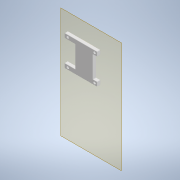
# Autodesk Inventor part: OLED
Saved by Autodesk Inventor 2021 (Build 250183000, 183)
## iProperties
Created: 2022-09-01
Part Number: OLED
Material: Generic
Document SubType Name: Modeling
Designer: cmzgt
Density: 1 g/cm^3
Appearance: Default
Author: cmzgt
Autodesk Inventor part; units mm, degrees
ref_plane "YZ Plane" through (0, 0, 0) normal (1, 0, 0) x (0, 1, 0)
ref_plane "XZ Plane" through (0, 0, 0) normal (0, 1, 0) x (-1, 0, 0)
ref_plane "XY Plane" through (0, 0, 0) normal (0, 0, 1) x (1, 0, 0)
ref_plane "Work Plane1" through (0, 0, 0) normal (0, 0, 1) x (1, 0, 0)
sketch "Sketch1" plane through (0, 0, 0) normal (0, 0, 1) x (1, 0, 0)
  line L0 (26.085, -12.7501) -> (26.085, -38.7501) projected
  line L1 (15.085, -12.7501) -> (26.085, -12.7501) projected
  line L2 (15.085, -38.7501) -> (15.085, -12.7501) projected
  line L3 (26.085, -38.7501) -> (15.085, -38.7501) projected
  line L4 (26.085, -25.7501) -> (15.085, -25.7501)
  line L5 (20.585, -38.7501) -> (20.585, -12.7501)
  line L6 (15.2194, -38.2641) -> (25.9506, -38.2641)
  line L7 (25.9506, -38.2641) -> (25.9506, -13.236)
  line L8 (25.9506, -13.236) -> (15.2194, -13.236)
  line L9 (15.2194, -13.236) -> (15.2194, -38.2641)
  line L10 (15.2194, -38.2641) -> (25.9506, -13.236) construction
  line L11 (25.9506, -38.2641) -> (15.2194, -13.236) construction
  point P0 (0, 0)
  point P1 (20.585, -25.7501)
  constraints: 16 end point, 7 midpoint, 2 parallel, 1 horizontal, 1 perpendicular
extrude "Extrusion1" add sketch "Sketch1" against normal blind 1 contours L7 L6 L5 L4 | L4 L5 L8 L7 | L5 L4 L9 L8 | L5 L6 L9 L4
sketch "Sketch2" plane through (0, 0, 0) normal (0, 0, 1) x (1, 0, 0)
  line L0 (15.2194, -13.236) -> (15.2194, -38.2641) projected
  line L1 (15.2194, -38.2641) -> (25.9506, -38.2641) projected
  line L2 (25.9506, -38.2641) -> (25.9506, -13.236) projected
  line L3 (25.9506, -13.236) -> (15.2194, -13.236) projected
  line L4 (13.1635, -39.268) -> (28.9935, -39.268)
  line L5 (28.9935, -39.268) -> (28.9935, -12.2321)
  line L6 (28.9935, -12.2321) -> (13.1635, -12.2321)
  line L7 (13.1635, -12.2321) -> (13.1635, -39.268)
  line L8 (13.1635, -39.268) -> (28.9935, -12.2321) construction
  line L9 (28.9935, -39.268) -> (13.1635, -12.2321) construction
  line L10 (28.9935, -12.2321) -> (32.8035, -12.2321)
  line L11 (32.8035, -12.2321) -> (32.8035, -16.0421)
  line L12 (32.8035, -16.0421) -> (28.9935, -16.0421)
  line L13 (28.9935, -39.268) -> (32.8035, -39.268)
  line L14 (32.8035, -39.268) -> (32.8035, -35.458)
  line L15 (32.8035, -35.458) -> (28.9935, -35.458)
  line L16 (13.1635, -12.2321) -> (3.8747, -12.2321)
  line L17 (3.8747, -12.2321) -> (3.8747, -16.0421)
  line L18 (3.8747, -16.0421) -> (13.1635, -16.0421)
  line L19 (13.1635, -39.268) -> (3.8747, -39.268)
  line L20 (3.8747, -39.268) -> (3.8747, -35.458)
  line L21 (3.8747, -35.458) -> (13.1635, -35.458)
  circle A0 centre (30.455, -14.1001) radius 1 projected
  circle A1 centre (30.455, -37.4001) radius 1 projected
  circle A2 centre (6.655, -37.4001) radius 1 projected
  circle A3 centre (6.655, -14.1001) radius 1 projected
  point P0 (0, 0)
  point P1 (21.0785, -25.7501)
  dimension "d2" = 3.81
  dimension "d3" = 3.81
  dimension "d4" = 3.81
  dimension "d5" = 3.81
  dimension "d6" = 6.0858
  dimension "d7" = 4.1119
  dimension "d8" = 27.0359
  dimension "d9" = 3.81
  dimension "d10" = 3.81
  dimension "d11" = 2.0078
  dimension "d12" = 44.1517
  constraints: 36 end point, 8 perpendicular, 7 point on line, 3 horizontal, 3 parallel, 2 midpoint
  measures "d2" distance of L5.end L10.end
  measures "d3" distance of L10.end L11.end
  measures "d4" distance of L13.end L14.end
  measures "d5" distance of L14.end L15.end
  measures "d6" diameter of L5 L2
  measures "d7" diameter of L7 L0
  measures "d8" distance between parallel lines of L6 L4
  measures "d9" distance of L16.end L17.end
  measures "d10" distance of L19.end L20.end
  measures "d11" diameter of L10 L3
  measures "d12" diameter of L20 L2
extrude "Extrusion2" add sketch "Sketch2" along normal blind 3 contours L3 L2 L1 L0 | L7 L6 L5 L4 | L19 L20 L21 L7 | L5 L15 L14 L13 | L18 L17 L16 L7 | L5 L10 L11 L12
fillet "Fillet1" radius 0.3175 30 edges at (32.8035, -16.0421, 1.5) (32.8035, -12.2321, 1.5) (30.8985, -16.0421, 3) (18.3391, -12.2321, 3) (28.9935, -25.7501, 3) (28.9935, -16.0421, 1.5) (30.8985, -16.0421, 0) (28.9935, -25.7501, 0) (32.8035, -35.458, 1.5) (30.8985, -35.458, 3) (18.3391, -39.268, 3) (32.8035, -39.268, 1.5) (32.8035, -37.363, 3) (32.8035, -14.1371, 3) (28.9935, -35.458, 1.5) (30.8985, -35.458, 0) (18.3391, -39.268, 0) (3.8747, -39.268, 1.5) (3.8747, -37.363, 3) (8.5191, -35.458, 3) (13.1635, -25.7501, 3) (8.5191, -16.0421, 3) (3.8747, -16.0421, 1.5) (3.8747, -14.1371, 3) (18.3391, -12.2321, 0) (3.8747, -12.2321, 1.5) (8.5191, -16.0421, 0) (8.5191, -35.458, 0) (32.8035, -37.363, 0) (32.8035, -14.1371, 0)
body "Solid1"
